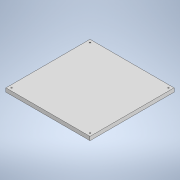
# Autodesk Inventor part: bakeoutbox lid
Saved by Autodesk Inventor 2020.2 (Build 242310000, 310)
## iProperties
Created: 2020-02-04
Part Number: bakeoutbox lid
Material: Generic
Document SubType Name: Modeling
Designer: ColinP
Density: 1 g/cm^3
Appearance: Default
Author: ColinP
Autodesk Inventor part; units mm, degrees
ref_plane "YZ Plane" through (0, 0, 0) normal (1, 0, 0) x (0, 1, 0)
ref_plane "XZ Plane" through (0, 0, 0) normal (0, 1, 0) x (-1, 0, 0)
ref_plane "XY Plane" through (0, 0, 0) normal (0, 0, 1) x (1, 0, 0)
sketch "Sketch1" plane through (0, 0, 0) normal (0, 1, 0) x (-1, 0, 0)
  line L0 (112.5, 112.5) -> (-112.5, 112.5)
  line L1 (-112.5, 112.5) -> (-112.5, -112.5)
  line L2 (-112.5, -112.5) -> (112.5, -112.5)
  line L3 (112.5, -112.5) -> (112.5, 112.5)
  point P0 (0, 0)
  dimension "d0" = 225
  dimension "d1" = 225
  constraints: 8 end point, 2 parallel, 1 horizontal, 1 perpendicular
  measures "d0" distance of L2.end L1.end
  measures "d1" distance of L1.end L0.end
extrude "Extrusion1" add sketch "Sketch1" along normal blind 10
sketch "Sketch2" plane through (0, 10, 0) normal (0, 1, 0) x (1, 0, 0)
  line L0 (-112.5, -112.5) -> (112.5, -112.5) projected
  line L1 (112.5, -112.5) -> (112.5, -105)
  line L2 (112.5, -112.5) -> (112.5, 112.5) projected
  line L3 (112.5, -105) -> (105, -105)
  line L4 (105, -105) -> (105, 105)
  line L5 (105, 105) -> (-105, 105)
  line L6 (-105, 105) -> (-105, -105)
  line L7 (-105, -105) -> (105, -105)
  point P0 (0, 0)
  dimension "d4" = 7.5
  dimension "d5" = 7.5
  dimension "d6" = 210
  dimension "d7" = 90
  dimension "d8" = 210
  dimension "d9" = 90
  dimension "d10" = 210
  dimension "d11" = 90
  constraints: 12 end point, 4 perpendicular, 1 point on line
  measures "d4" distance of L0.end L1.end
  measures "d5" distance of L1.end L3.end
  measures "d6" distance of L3.end L4.end
  measures "d7" angle of L3 L4
  measures "d8" distance of L4.end L5.end
  measures "d9" angle of L5 L4
  measures "d10" distance of L5.end L6.end
  measures "d11" angle of L6 L5
hole "Hole1" at (-105, 10, 105) at (-105, 10, -105) at (105, 10, -105) at (105, 10, 105) direction (0, -1, 0) diameter 3.302 depth 12.3 thread size "8-32 UNC" class "2B" standard "ANSI Unified Screw Threads"
body "Solid1"
